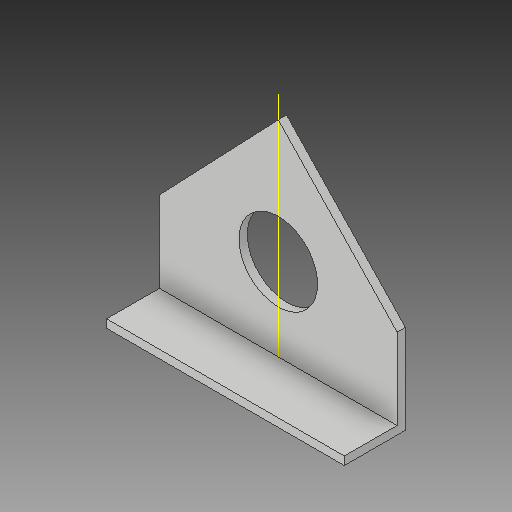
# Autodesk Inventor part: rsSnowBlowerMount
Saved by Autodesk Inventor 2017 (Build 210142000, 142)
## iProperties
Created: 2016-02-01
Part Number: rsSnowBlowerMount
Material: Generic
Document SubType Name: Modeling
Designer: steele
Density: 1 g/cm^3
Appearance: Default
Mass: 28.3152 g
Surface Area: 191.707 cm^2
Volume: 28.3152 cm^3
Author: steele
Autodesk Inventor part; units mm, degrees
ref_plane "YZ Plane" through (0, 0, 0) normal (1, 0, 0) x (0, 1, 0)
ref_plane "XZ Plane" through (0, 0, 0) normal (0, 1, 0) x (-1, 0, 0)
ref_plane "XY Plane" through (0, 0, 0) normal (0, 0, 1) x (1, 0, 0)
sketch "Sketch1" plane through (0, 0, 0) normal (0, 0, 1) x (1, 0, 0)
  line L0 (0, 0) -> (45.72, 0)
  line L1 (45.72, 0) -> (45.72, 34.29)
  line L2 (0, 0) -> (0, 82.169) construction
  line L3 (45.72, 34.29) -> (0, 82.169)
  line L4 (0, 0) -> (-45.72, 0)
  line L5 (-45.72, 0) -> (-45.72, 34.29)
  line L6 (-45.72, 34.29) -> (0, 82.169)
  dimension "d0" = 82.169
  dimension "d1" = 45.72
  dimension "d2" = 34.29
  constraints: 14 end point, 2 symmetric about line, 1 horizontal, 1 perpendicular, 1 vertical
  measures "d0" distance of L0.start L2.end
  measures "d1" distance of L0.start L0.end
  measures "d2" distance of L0.end L1.end
extrude "Extrusion1" add sketch "Sketch1" against normal blind 3.175
sketch "Sketch2" plane through (0, 0, 0) normal (0, 0, 1) x (1, 0, 0)
  line L0 (-45.72, 0) -> (-45.72, 34.29) projected
  line L1 (-45.72, 0) -> (45.72, 0)
  line L2 (45.72, 0) -> (45.72, 3.175)
  line L3 (45.72, 3.175) -> (-45.72, 3.175)
  line L4 (-45.72, 3.175) -> (-45.72, 0)
  point P0 (0, 0)
  dimension "d5" = 3.175
  constraints: 8 end point, 2 parallel, 1 horizontal, 1 perpendicular
  measures "d5" distance between parallel lines of L3 L1
extrude "Extrusion2" add sketch "Sketch2" along normal blind 20.32
sketch "Sketch3" plane through (0, 0, 0) normal (0, 0, 1) x (1, 0, 0)
  circle A0 centre (0, 34.925) radius 15.113
  line L0 (-45.72, 0) -> (45.72, 0) projected
  point P0 (0, 0)
  dimension "d8" = 30.226
  dimension "d9" = 34.925
  constraints: 1 centre point
  measures "d8" diameter of A0
  measures "d9" distance from line of A0.centre L0
extrude "Extrusion3" cut sketch "Sketch3" against normal through all
body "Solid1"
